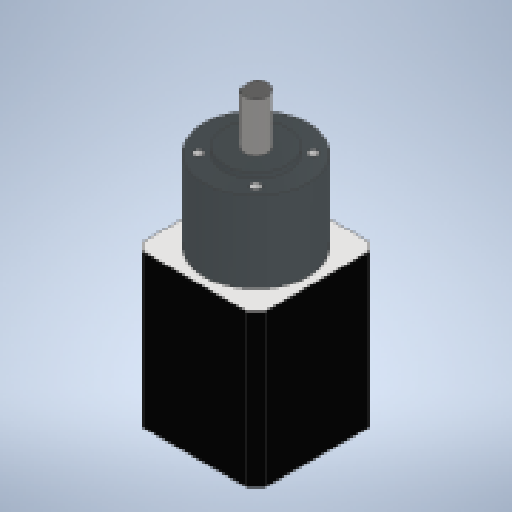
# Autodesk Inventor part: stepper 42-27
Saved by Autodesk Inventor 2025 (Build 290162000, 162)
## iProperties
Created: 2025-04-03
Part Number: stepper 42-27
Material: 一般
Document SubType Name: Modeling
Designer: gavin
Density: 1 g/cm^3
Appearance: 預設
Author: gavin
Autodesk Inventor part; units mm, degrees
ref_plane "YZ Plane" through (0, 0, 0) normal (1, 0, 0) x (0, 1, 0)
ref_plane "XZ Plane" through (0, 0, 0) normal (0, 1, 0) x (-1, 0, 0)
ref_plane "XY Plane" through (0, 0, 0) normal (0, 0, 1) x (1, 0, 0)
sketch "草圖1" plane through (0, 0, 0) normal (0, 1, 0) x (-1, 0, 0)
  line L0 (18, 21) -> (-18, 21)
  line L1 (-21, 18) -> (-21, -18)
  line L2 (-18, -21) -> (18, -21)
  line L3 (21, -18) -> (21, 18)
  line L4 (21, 21) -> (-21, -21) construction
  line L5 (-21, 21) -> (21, -21) construction
  line L6 (21, -18) -> (18, -21)
  line L7 (-18, -21) -> (-21, -18)
  line L8 (-21, 18) -> (-18, 21)
  line L9 (18, 21) -> (21, 18)
  point P0 (0, 0)
  dimension "d0" = 42
  dimension "d1" = 42
  dimension "d2" = 3
  dimension "d3" = 3
  dimension "d4" = 3
  dimension "d5" = 3
  dimension "d6" = 3
  dimension "d7" = 3
  dimension "d8" = 3
  dimension "d9" = 3
  constraints: 20 end point, 8 point on line, 2 midpoint, 2 parallel, 1 horizontal, 1 perpendicular
  measures "d0" distance of L5.end L4.end
  measures "d1" distance of L4.end L5.start
  measures "d2" distance of L3.start L5.end
  measures "d3" distance of L2.end L5.end
  measures "d4" distance of L2.start L4.end
  measures "d5" distance of L1.end L4.end
  measures "d6" distance of L1.start L5.start
  measures "d7" distance of L0.end L5.start
  measures "d8" distance of L0.start L4.start
  measures "d9" distance of L3.end L4.start
extrude "擠出1" add sketch "草圖1" along normal blind 52.6
sketch "草圖2" plane through (0, 52.6, 0) normal (0, 1, 0) x (1, 0, 0)
  circle A0 centre (0, 0) radius 18
  dimension "d12" = 36
  constraints: 1 centre point, 1 coincident
  measures "d12" diameter of A0
extrude "擠出2" add sketch "草圖2" along normal blind 28
sketch "草圖3" plane through (0, 80.6, 0) normal (0, 1, 0) x (1, 0, 0)
  circle A0 centre (0, 0) radius 14 construction
  circle A1 centre (0, 0) radius 11
  line L0 (0, 0) -> (-19.5, -19.5) construction
  line L1 (-21, -18) -> (-18, -21) projected
  circle A2 centre (-9.8995, -9.8995) radius 1.5
  circle A3 centre (9.8995, -9.8995) radius 1.5
  circle A4 centre (9.8995, 9.8995) radius 1.5
  circle A5 centre (-9.8995, 9.8995) radius 1.5
  dimension "d15" = 28
  dimension "d16" = 22
  dimension "d18" = 3
  dimension "d21" = 360
  constraints: 5 centre point, 3 coincident, 2 end point, 1 midpoint, 1 point on line, 12 other
  measures "d16" diameter of A1
  measures "d18" diameter of A2
extrude "擠出3" cut sketch "草圖3" against normal blind 6 contours A2 | A3 | A4 | A5
extrude "擠出4" add sketch "草圖3" along normal blind 2 contours A1
sketch "草圖4" plane through (0, 82.6, 0) normal (0, 1, 0) x (1, 0, 0)
  circle A0 centre (0, 0) radius 4
  dimension "d27" = 8
  constraints: 1 centre point, 1 coincident
  measures "d27" diameter of A0
extrude "擠出5" add sketch "草圖4" along normal blind 17
sketch "草圖5" plane through (0, 99.6, 0) normal (0, 1, 0) x (1, 0, 0)
  circle A0 centre (0, 0) radius 4 projected
  line L0 (-3, -2.6458) -> (-3, 2.6458)
  dimension "d30" = 7
  constraints: 2 end point, 2 point on circle, 1 vertical
extrude "擠出6" cut sketch "草圖5" against normal blind 15 contours L0 A0 picked at (-3.1815, -0.6179)
sketch "草圖7" plane through (0, 0, 0) normal (0, -1, 0) x (1, 0, 0)
  point P0 (0, 0)
  point P1 (0, 0)
  constraints: 1 coincident
equation "\"d3\" = d2"
equation "\"d4\" = d2"
equation "\"d5\" = d4"
equation "\"d6\" = d2"
equation "\"d7\" = d6"
equation "\"d8\" = d2"
equation "\"d9\" = d8"
